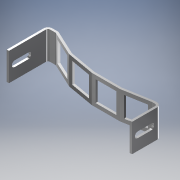
# Autodesk Inventor part: key_holder_metal
Saved by Autodesk Inventor 2018 (Build 220112000, 112)
## iProperties
Created: 2018-04-04
Part Number: key_holder_metal
Material: アルミニウム 6061
Document SubType Name: Sheet Metal
Designer: NaMACHAN
Density: 2.7 g/cm^3
Sheet Metal Rule: Default_mm
Appearance: アルミニウム - フラット
Author: NaMACHAN
Autodesk Inventor part; units mm, degrees
ref_plane "YZ Plane" through (0, 0, 0) normal (1, 0, 0) x (0, 1, 0)
ref_plane "XZ Plane" through (0, 0, 0) normal (0, 1, 0) x (-1, 0, 0)
ref_plane "XY Plane" through (0, 0, 0) normal (0, 0, 1) x (1, 0, 0)
sketch "スケッチ2" plane through (0, 0, 0) normal (0, 1, 0) x (-1, 0, 0)
  line L0 (-9.5, -9.5) -> (9.5, -9.5)
  line L1 (9.5, -9.5) -> (9.5, 9.5)
  line L2 (9.5, 9.5) -> (-9.5, 9.5)
  line L3 (-9.5, 9.5) -> (-9.5, -9.5)
  line L4 (-9.5, -9.5) -> (9.5, 9.5) construction
  line L5 (9.5, -9.5) -> (-9.5, 9.5) construction
  point P0 (0, 0)
  dimension "d4" = 19
  dimension "d5" = 19
  measures "d4" distance of L2.end L1.end
  measures "d5" distance of L1.end L0.end
extrude "プレート1" add sketch "スケッチ2" along normal blind 1.5
sketch "スケッチ3" plane through (9.2395, 1.4772, -9.5) normal (0.1736482, -0.9848078, 0) x (0.9848078, 0.1736482, 0)
  line L0 (0, 19) -> (0, 0)
  line L1 (0, 0) -> (19, 0)
  line L2 (19, 0) -> (19, 19)
  line L3 (19, 19) -> (0, 19)
  constraints: 6 end point, 1 horizontal, 1 perpendicular, 1 vertical
edge flange "フランジ1" height 19 angle 10 thickness 1.5 bend radius 1.5 thickness toward (0.1736482, -0.9848078, 0) relief straight relief width 1.5 relief depth 0.75 edges at (9.5, 1.5, 0) wall of the first edge with corners at (9.2395, 1.4772, 9.5) (9.2395, 1.4772, -9.5) (27.9509, 4.7765, -9.5) (27.9509, 4.7765, 9.5)
bend "曲げ1"
corner "コーナー1"
sketch "スケッチ4" plane through (-9.2395, 1.4772, 9.5) normal (-0.1736482, -0.9848078, 0) x (0.9848078, -0.1736482, 0)
  line L0 (0, -19) -> (0, 0)
  line L1 (0, 0) -> (-19, 0)
  line L2 (-19, 0) -> (-19, -19)
  line L3 (-19, -19) -> (0, -19)
  constraints: 6 end point, 1 horizontal, 1 perpendicular, 1 vertical
edge flange "フランジ2" height 19 angle 10 thickness 1.5 bend radius 1.5 thickness toward (-0.1736482, -0.9848078, 0) relief straight relief width 1.5 relief depth 0.75 edges at (-9.5, 1.5, 0) wall of the first edge with corners at (-9.2395, 1.4772, -9.5) (-9.2395, 1.4772, 9.5) (-27.9509, 4.7765, 9.5) (-27.9509, 4.7765, -9.5)
bend "曲げ2"
corner "コーナー2"
sketch "スケッチ5" plane through (-27.5774, 4.6588, 9.5) normal (-0.4226183, -0.9063078, 0) x (0.9063078, -0.4226183, 0)
  line L0 (0, -19) -> (0, 0)
  line L1 (0, 0) -> (-19.1975, 0)
  line L2 (-19.1975, 0) -> (-19.1975, -19)
  line L3 (-19.1975, -19) -> (0, -19)
  constraints: 6 end point, 1 horizontal, 1 perpendicular, 1 vertical
edge flange "フランジ3" height 19 angle 15 thickness 1.5 bend radius 1.5 thickness toward (-0.4226183, -0.9063078, 0) relief straight relief width 1.5 relief depth 0.75 edges at (-27.9509, 4.7765, 0) wall of the first edge with corners at (-27.5774, 4.6588, -9.5) (-27.5774, 4.6588, 9.5) (-44.9762, 12.772, 9.5) (-44.9762, 12.772, -9.5)
bend "曲げ3"
corner "コーナー3"
sketch "スケッチ6" plane through (27.9509, 3.2765, -9.5) normal (0, 1, 0) x (1, 0, 0)
  line L0 (0, 19) -> (0, 0)
  line L1 (0, 0) -> (5, 0)
  line L2 (5, 0) -> (5, 19)
  line L3 (5, 19) -> (0, 19)
  constraints: 6 end point, 1 horizontal, 1 perpendicular, 1 vertical
edge flange "フランジ4" height 5 angle -10 thickness 1.5 bend radius 1.5 thickness toward (0, 1, 0) relief straight relief width 1.5 relief depth 0.75 edges at (27.9509, 4.7765, 0) wall of the first edge with corners at (27.9509, 3.2765, 9.5) (27.9509, 3.2765, -9.5) (32.9509, 3.2765, -9.5) (32.9509, 3.2765, 9.5)
bend "曲げ4"
corner "コーナー4"
sketch "スケッチ7" plane through (31.4509, 4.7765, -9.5) normal (1, 0, 0) x (0, -1, 0)
  line L0 (0, 19) -> (0, 0)
  line L1 (0, 0) -> (20, 0)
  line L2 (20, 0) -> (20, 19)
  line L3 (20, 19) -> (0, 19)
  constraints: 6 end point, 1 horizontal, 1 perpendicular, 1 vertical
edge flange "フランジ5" height 20 angle -90 thickness 1.5 bend radius 1.5 thickness toward (1, 0, 0) relief straight relief width 1.5 relief depth 0.75 edges at (32.9509, 4.7765, 0) wall of the first edge with corners at (31.4509, 4.7765, 9.5) (31.4509, 4.7765, -9.5) (31.4509, -15.2235, -9.5) (31.4509, -15.2235, 9.5)
bend "曲げ5"
corner "コーナー5"
sketch "スケッチ8" plane through (-44.9762, 11.272, 9.5) normal (0, 1, 0) x (1, 0, 0)
  line L0 (0, -19) -> (0, 0)
  line L1 (0, 0) -> (-7.073, 0)
  line L2 (-7.073, 0) -> (-7.073, -19)
  line L3 (-7.073, -19) -> (0, -19)
  constraints: 6 end point, 1 horizontal, 1 perpendicular, 1 vertical
edge flange "フランジ6" height 7.073 angle -25 thickness 1.5 bend radius 1.5 thickness toward (0, 1, 0) relief straight relief width 1.5 relief depth 0.75 edges at (-44.9762, 12.772, 0) wall of the first edge with corners at (-44.9762, 11.272, -9.5) (-44.9762, 11.272, 9.5) (-52.0492, 11.272, 9.5) (-52.0492, 11.272, -9.5)
bend "曲げ6"
corner "コーナー6"
sketch "スケッチ10" plane through (-50.5492, 12.772, 9.5) normal (-1, 0, 0) x (0, 1, 0)
  line L0 (0, -19) -> (0, 0)
  line L1 (0, 0) -> (-27.995, 0)
  line L2 (-27.995, 0) -> (-27.995, -19)
  line L3 (-27.995, -19) -> (0, -19)
  constraints: 6 end point, 1 horizontal, 1 perpendicular, 1 vertical
edge flange "フランジ8" height 27.995 angle -90 thickness 1.5 bend radius 1.5 thickness toward (-1, 0, 0) relief straight relief width 1.5 relief depth 0.75 edges at (-52.0492, 12.772, 0) wall of the first edge with corners at (-50.5492, 12.772, -9.5) (-50.5492, 12.772, 9.5) (-50.5492, -15.223, 9.5) (-50.5492, -15.223, -9.5)
bend "曲げ8"
corner "コーナー8"
sketch "スケッチ11" plane through (9.498, 1.5228, 9.5) normal (-0.1736482, 0.9848078, 0) x (0.9848078, 0.1736482, 0)
  line L0 (2.2375, 16.5) -> (16.2375, 16.5)
  line L1 (16.2375, 16.5) -> (16.2375, 2.5)
  line L2 (16.2375, 2.5) -> (2.2375, 2.5)
  line L3 (2.2375, 2.5) -> (2.2375, 16.5)
  line L4 (2.2375, 16.5) -> (16.2375, 2.5) construction
  line L5 (16.2375, 16.5) -> (2.2375, 2.5) construction
  line L6 (20.4467, 19) -> (20.4467, 0) projected
  line L7 (18.4751, 0) -> (0, 0) projected
  point P0 (-9.6181, 9.5)
  point P1 (9.2375, 9.5)
  point P2 (9.2375, 9.5)
  point P3 (20.4467, 9.5)
  point P4 (9.2375, 9.5)
  point P5 (9.2375, 0)
  dimension "d87" = 14
  dimension "d88" = 14
  constraints: 12 end point, 6 midpoint, 2 parallel, 1 horizontal, 1 horizontal alignment, 1 perpendicular, 1 vertical alignment
  measures "d87" distance of L1.end L2.end
  measures "d88" distance of L0.end L1.end
extrude "押し出し2" cut sketch "スケッチ11" against normal blind 1.5
sketch "スケッチ12" plane through (0, 1.5, 0) normal (0, 1, 0) x (1, 0, 0)
  line L0 (-7, 7) -> (7, 7)
  line L1 (7, 7) -> (7, -7)
  line L2 (7, -7) -> (-7, -7)
  line L3 (-7, -7) -> (-7, 7)
  line L4 (-7, 7) -> (7, -7) construction
  line L5 (7, 7) -> (-7, -7) construction
  point P0 (0, 0)
  dimension "d91" = 14
  dimension "d92" = 14
  constraints: 12 end point, 2 midpoint, 2 parallel, 1 horizontal, 1 perpendicular
  measures "d91" distance of L1.end L2.end
  measures "d92" distance of L0.end L1.end
extrude "押し出し3" cut sketch "スケッチ12" against normal blind 1.5
sketch "スケッチ13" plane through (-9.498, 1.5228, 9.5) normal (0.1736482, 0.9848078, 0) x (0.9848078, -0.1736482, 0)
  line L0 (-2.1713, 16.5) -> (-16.1713, 16.5)
  line L1 (-16.1713, 16.5) -> (-16.1713, 2.5)
  line L2 (-16.1713, 2.5) -> (-2.1713, 2.5)
  line L3 (-2.1713, 2.5) -> (-2.1713, 16.5)
  line L4 (-2.1713, 16.5) -> (-16.1713, 2.5) construction
  line L5 (-16.1713, 16.5) -> (-2.1713, 2.5) construction
  line L6 (-18.3426, 19) -> (0, 19) projected
  line L7 (0.2605, 19) -> (0.2605, 0) projected
  point P0 (9.6181, 9.5)
  point P1 (-9.1713, 9.5)
  point P2 (-9.1713, 9.5)
  point P3 (-2.1713, 9.5)
  point P4 (-9.1713, 9.5)
  point P5 (-9.1713, 19)
  point P6 (0.2605, 9.5)
  dimension "d95" = 14
  dimension "d96" = 14
  constraints: 12 end point, 7 midpoint, 2 horizontal alignment, 2 parallel, 1 horizontal, 1 perpendicular, 1 vertical alignment
  measures "d95" distance of L2.end L1.end
  measures "d96" distance of L1.end L0.end
extrude "押し出し4" cut sketch "スケッチ13" against normal blind 1.5
sketch "スケッチ14" plane through (-27.9354, 4.8257, 9.5) normal (0.4226183, 0.9063078, 0) x (0.9063078, -0.4226183, 0)
  line L0 (-2.0687, 16.5) -> (-16.0687, 16.5)
  line L1 (-16.0687, 16.5) -> (-16.0687, 2.5)
  line L2 (-16.0687, 2.5) -> (-2.0687, 2.5)
  line L3 (-2.0687, 2.5) -> (-2.0687, 16.5)
  line L4 (-2.0687, 16.5) -> (-16.0687, 2.5) construction
  line L5 (-16.0687, 16.5) -> (-2.0687, 2.5) construction
  line L6 (-18.1374, 19) -> (0, 19) projected
  line L7 (0, 0) -> (0, 19) projected
  point P0 (27.3575, 9.5)
  point P1 (-9.0687, 9.5)
  point P2 (-9.0687, 9.5)
  point P3 (-9.0687, 19)
  point P4 (-9.0687, 9.5)
  point P5 (0, 9.5)
  dimension "d99" = 14
  dimension "d100" = 14
  constraints: 12 end point, 6 midpoint, 2 parallel, 1 horizontal, 1 horizontal alignment, 1 perpendicular, 1 vertical alignment
  measures "d99" distance of L2.end L1.end
  measures "d100" distance of L1.end L0.end
extrude "押し出し5" cut sketch "スケッチ14" against normal blind 1.5
sketch "スケッチ17" plane through (32.9509, -15.2235, 9.5) normal (1, 0, 0) x (0, 0, -1)
  line L0 (0, 0) -> (19, 0) projected
  line L1 (0, 17) -> (0, 0) projected
  line L2 (19, 17) -> (19, 0) projected
  arc A0 (11.4998, 13.0278) -> (7.5, 13) centre (9.5, 13) ccw
  line L3 (11.4998, 13.0278) -> (11.4998, 4)
  arc A1 (7.5, 4) -> (11.4998, 4) centre (9.4999, 4) ccw
  line L4 (7.5, 4) -> (7.5, 13)
  line L5 (19, 17) -> (0, 17) projected
  point P0 (9.5, 15.2235)
  point P1 (9.5, 0)
  dimension "d129" = 2
  dimension "d130" = 1.9999
  dimension "d131" = 4
  dimension "d132" = 4
  constraints: 4 end point, 4 point on circle, 3 tangent, 2 centre point, 1 midpoint, 1 parallel, 1 vertical, 1 vertical alignment
  measures "d129" radius of A0
  measures "d130" radius of A1
  measures "d131" distance from line of L5 A0.centre
  measures "d132" distance from line of L0 A1.centre
extrude "押し出し7" cut sketch "スケッチ17" against normal blind 100 contours L3 A1 L4 A0
equation "\"d6\" = Thickness"
equation "\"d7\" = BendReliefWidth"
equation "\"d8\" = BendReliefDepth"
equation "\"d9\" = MinimumRemnant"
equation "\"d10\" = TransitionRadius"
equation "\"d13\" = BendRadius"
equation "\"d14\" = CornerReliefSize"
equation "\"d15\" = GapSize"
equation "\"d16\" = JacobiRadiusSize"
equation "\"d17\" = BendReliefWidth"
equation "\"d18\" = BendReliefDepth"
equation "\"d19\" = MinimumRemnant"
equation "\"d20\" = TransitionRadius"
equation "\"d23\" = BendRadius"
equation "\"d24\" = CornerReliefSize"
equation "\"d25\" = GapSize"
equation "\"d26\" = JacobiRadiusSize"
equation "\"d27\" = BendReliefWidth"
equation "\"d28\" = BendReliefDepth"
equation "\"d29\" = MinimumRemnant"
equation "\"d30\" = TransitionRadius"
equation "\"d33\" = BendRadius"
equation "\"d34\" = CornerReliefSize"
equation "\"d35\" = GapSize"
equation "\"d36\" = JacobiRadiusSize"
equation "\"d37\" = BendReliefWidth"
equation "\"d38\" = BendReliefDepth"
equation "\"d39\" = MinimumRemnant"
equation "\"d40\" = TransitionRadius"
equation "\"d43\" = BendRadius"
equation "\"d44\" = CornerReliefSize"
equation "\"d45\" = GapSize"
equation "\"d46\" = JacobiRadiusSize"
equation "\"d47\" = BendReliefWidth"
equation "\"d48\" = BendReliefDepth"
equation "\"d49\" = MinimumRemnant"
equation "\"d50\" = TransitionRadius"
equation "\"d53\" = BendRadius"
equation "\"d54\" = CornerReliefSize"
equation "\"d55\" = GapSize"
equation "\"d56\" = JacobiRadiusSize"
equation "\"d57\" = BendReliefWidth"
equation "\"d58\" = BendReliefDepth"
equation "\"d59\" = MinimumRemnant"
equation "\"d60\" = TransitionRadius"
equation "\"d63\" = BendRadius"
equation "\"d64\" = CornerReliefSize"
equation "\"d65\" = GapSize"
equation "\"d66\" = JacobiRadiusSize"
equation "\"d77\" = BendReliefWidth"
equation "\"d78\" = BendReliefDepth"
equation "\"d79\" = MinimumRemnant"
equation "\"d80\" = TransitionRadius"
equation "\"d83\" = BendRadius"
equation "\"d84\" = CornerReliefSize"
equation "\"d85\" = GapSize"
equation "\"d86\" = JacobiRadiusSize"
equation "\"BendRadius\" = Thickness"
equation "\"BendReliefWidth\" = Thickness"
equation "\"BendReliefDepth\" = 0.5 * Thickness"
equation "\"CornerReliefSize\" = 4 * Thickness"
equation "\"MinimumRemnant\" = 2 * Thickness"
equation "\"TransitionRadius\" = BendRadius"
equation "\"JacobiRadiusSize\" = BendRadius"
equation "\"GapSize\" = Thickness"
equation "\"Thickness\" = 1.5"
